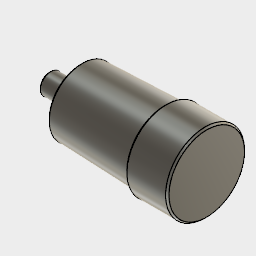
Part B (Autodesk Fusion 360 design; units mm, degrees)
Autodesk Fusion 360 part; units mm, degrees
sketch "Sketch1" plane through (0, 0, 0) normal (0, 1, 0) x (1, 0, 0)
  line L0 (0, 0) -> (0, -10.033)
  line L1 (25.4, -10.92) -> (25.4, -11.938)
  line L2 (25.4, -11.938) -> (38.1, -11.938)
  line L3 (38.1, -11.938) -> (38.1, 0)
  line L4 (38.1, 0) -> (0, 0)
  line L5 (25.4, -10.92) -> (0, -10.033)
  line L6 (0, -3.175) -> (-9.525, -3.175)
  line L7 (-9.525, -3.175) -> (-9.525, 0)
  line L8 (-9.525, 0) -> (0, 0)
  dimension "d1" = 10.033
  dimension "d2" = 25.4
  dimension "d3" = 12.7
  dimension "d4" = 11.938
  dimension "d5" = 92
  dimension "d7" = 3.175
  dimension "d8" = 9.525
  measures "d1" distance of L0.start L0.end
  measures "d2" distance of L0.end L1.start
  measures "d3" distance of L1.end L2.end
  measures "d4" distance of L2.end L3.end
  measures "d5" angle of L0 L5
  measures "d7" distance of L6.end L7.end
  measures "d8" distance of L6.start L6.end
revolve "Revolve1" add sketch "Sketch1" angle 360 about axis through (38.1, 0, 0) along (-1, 0, 0)
chamfer "Chamfer1" distance 0.508 angle 45 5 edges at (-9.525, -1.1481, -2.9601) (0, -1.1481, -2.9601) (0, -3.6281, -9.354) (25.4, -4.317, -11.1301) (38.1, -4.317, -11.1301)
